Autodesk Fusion 360 part; units mm, degrees
(part 9 of 20)
  spline S703 degree 3 poles (18.7258, -338.1357) (18.7536, -338.279) (18.8048, -338.5439) (18.9786, -338.7491) (19.0584, -338.8434) knots 0 0 0 0 0.042908 0.079365 0.079365 0.079365 0.079365
  spline S704 degree 3 poles (19.0584, -338.8434) (19.1506, -338.9125) (19.3372, -339.0525) (19.5699, -339.0711) (19.6877, -339.0804) knots 0 0 0 0 0.033826 0.068485 0.068485 0.068485 0.068485
  spline S705 degree 3 poles (19.6877, -339.0804) (19.8301, -339.0661) (20.1169, -339.0374) (20.3305, -338.8437) (20.438, -338.7462) knots 0 0 0 0 0.041772 0.0841 0.0841 0.0841 0.0841
  spline S706 degree 3 poles (20.438, -338.7462) (20.5275, -338.6211) (20.7167, -338.3566) (20.7352, -338.031) (20.7449, -337.8594) knots 0 0 0 0 0.045186 0.095569 0.095569 0.095569 0.095569
  spline S707 degree 3 poles (20.7449, -337.8594) (20.7359, -337.6971) (20.7188, -337.3908) (20.5359, -337.1458) (20.4499, -337.0306) knots 0 0 0 0 0.047557 0.089725 0.089725 0.089725 0.089725
  spline S708 degree 3 poles (20.4499, -337.0306) (20.3414, -336.9421) (20.1168, -336.7589) (19.8271, -336.7379) (19.6774, -336.7271) knots 0 0 0 0 0.040971 0.08482 0.08482 0.08482 0.08482
  spline S709 degree 3 poles (19.6774, -336.7271) (19.5817, -336.7322) (19.3944, -336.7423) (19.2249, -336.8225) (19.1419, -336.8618) knots 0 0 0 0 0.028423 0.055689 0.055689 0.055689 0.055689
  spline S710 degree 3 poles (19.1419, -336.8618) (19.0671, -336.9094) (18.9202, -337.0026) (18.8172, -337.1427) (18.7667, -337.2114) knots 0 0 0 0 0.026342 0.051681 0.051681 0.051681 0.051681
  line L196 (18.7667, -337.2114) -> (18.1903, -337.1364)
  line L197 (18.1903, -337.1364) -> (18.6746, -334.5682)
  line L198 (18.6746, -334.5682) -> (21.161, -334.5681)
  line L199 (21.161, -334.5681) -> (21.161, -335.1548)
  line L200 (21.161, -335.1548) -> (19.1657, -335.1548)
  line L201 (19.1657, -335.1548) -> (18.8963, -336.4986)
  spline S711 degree 3 poles (18.8963, -336.4986) (19.0458, -336.4071) (19.3367, -336.2291) (19.6761, -336.1993) (19.8411, -336.1848) knots 0 0 0 0 0.051785 0.100763 0.100763 0.100763 0.100763
  spline S712 degree 3 poles (19.8411, -336.1848) (20.0503, -336.2032) (20.4659, -336.2397) (20.7868, -336.5061) (20.9461, -336.6384) knots 0 0 0 0 0.061424 0.122014 0.122014 0.122014 0.122014
  spline S713 degree 3 poles (20.9461, -336.6384) (21.0774, -336.8038) (21.3483, -337.1451) (21.38, -337.5805) (21.3964, -337.8048) knots 0 0 0 0 0.061868 0.12764 0.12764 0.12764 0.12764
  spline S714 degree 3 poles (21.3964, -337.8048) (21.3812, -338.0218) (21.3513, -338.4476) (21.1161, -338.8035) (21.0008, -338.9781) knots 0 0 0 0 0.064036 0.125703 0.125703 0.125703 0.125703
  spline S715 degree 3 poles (21.0008, -338.9781) (20.823, -339.1551) (20.46, -339.5168) (19.9487, -339.5621) (19.6877, -339.5852) knots 0 0 0 0 0.072854 0.148822 0.148822 0.148822 0.148822
  spline S716 degree 3 poles (19.6877, -339.5852) (19.4745, -339.5725) (19.0669, -339.5481) (18.7332, -339.3146) (18.5741, -339.2033) knots 0 0 0 0 0.062678 0.119794 0.119794 0.119794 0.119794
  spline S717 degree 3 poles (18.5741, -339.2033) (18.4455, -339.0629) (18.1812, -338.7745) (18.1151, -338.3885) (18.0812, -338.1903) knots 0 0 0 0 0.055877 0.114795 0.114795 0.114795 0.114795
  line L202 (29.6139, -389.4998) -> (29.6138, -385.8777)
  line L203 (29.6138, -385.8777) -> (30.163, -385.8777)
  line L204 (30.163, -385.8777) -> (30.163, -386.3859)
  spline S718 degree 3 poles (30.163, -386.3859) (30.2249, -386.3013) (30.3497, -386.1308) (30.5271, -386.0158) (30.6166, -385.9579) knots 0 0 0 0 0.031158 0.062835 0.062835 0.062835 0.062835
  spline S719 degree 3 poles (30.6166, -385.9579) (30.7157, -385.9106) (30.9196, -385.8135) (31.1453, -385.8018) (31.2612, -385.7958) knots 0 0 0 0 0.032617 0.067048 0.067048 0.067048 0.067048
  spline S720 degree 3 poles (31.2612, -385.7958) (31.3857, -385.8006) (31.6181, -385.8094) (31.825, -385.9143) (31.9211, -385.963) knots 0 0 0 0 0.036859 0.068796 0.068796 0.068796 0.068796
  spline S721 degree 3 poles (31.9211, -385.963) (32.0008, -386.0247) (32.1617, -386.1493) (32.2432, -386.336) (32.2844, -386.4302) knots 0 0 0 0 0.029725 0.060035 0.060035 0.060035 0.060035
  spline S722 degree 3 poles (32.2844, -386.4302) (32.4346, -386.2452) (32.7257, -385.8867) (33.1821, -385.8254) (33.4031, -385.7958) knots 0 0 0 0 0.068625 0.133023 0.133023 0.133023 0.133023
  spline S723 degree 3 poles (33.4031, -385.7958) (33.5681, -385.8042) (33.876, -385.8199) (34.1191, -386.0073) (34.2319, -386.0942) knots 0 0 0 0 0.048244 0.08997 0.08997 0.08997 0.08997
  spline S724 degree 3 poles (34.2319, -386.0942) (34.3161, -386.2166) (34.5056, -386.4915) (34.516, -386.8271) (34.5218, -387.0134) knots 0 0 0 0 0.043695 0.098195 0.098195 0.098195 0.098195
  line L205 (34.5218, -387.0134) -> (34.5218, -389.4997)
  line L206 (34.5218, -389.4997) -> (33.9113, -389.4998)
  line L207 (33.9113, -389.4998) -> (33.9113, -387.218)
  spline S725 degree 3 poles (33.9113, -387.218) (33.9112, -387.1118) (33.9112, -386.9325) (33.8688, -386.7586) (33.8516, -386.6877) knots 0 0 0 0 0.031711 0.053535 0.053535 0.053535 0.053535
  spline S726 degree 3 poles (33.8516, -386.6877) (33.8271, -386.636) (33.7773, -386.5306) (33.683, -386.4618) (33.635, -386.4268) knots 0 0 0 0 0.016863 0.034394 0.034394 0.034394 0.034394
  spline S727 degree 3 poles (33.635, -386.4268) (33.5793, -386.3979) (33.4638, -386.3382) (33.3339, -386.3314) (33.2666, -386.3279) knots 0 0 0 0 0.018597 0.038532 0.038532 0.038532 0.038532
  spline S728 degree 3 poles (33.2666, -386.3279) (33.1455, -386.3377) (32.9075, -386.3569) (32.7229, -386.5079) (32.6323, -386.582) knots 0 0 0 0 0.035532 0.069798 0.069798 0.069798 0.069798
  spline S729 degree 3 poles (32.6323, -386.582) (32.5589, -386.6887) (32.3918, -386.9318) (32.3842, -387.2288) (32.3799, -387.3954) knots 0 0 0 0 0.038079 0.086792 0.086792 0.086792 0.086792
  line L208 (32.3799, -387.3954) -> (32.3799, -389.4998)
  line L209 (32.3799, -389.4998) -> (31.766, -389.4998)
  line L210 (31.766, -389.4998) -> (31.766, -387.1464)
  spline S730 degree 3 poles (31.766, -387.1464) (31.7636, -387.0244) (31.7593, -386.8076) (31.6595, -386.6162) (31.6159, -386.5325) knots 0 0 0 0 0.036008 0.063954 0.063954 0.063954 0.063954
  spline S731 degree 3 poles (31.6159, -386.5325) (31.5537, -386.473) (31.4175, -386.3426) (31.2278, -386.3331) (31.1248, -386.3279) knots 0 0 0 0 0.025037 0.054812 0.054812 0.054812 0.054812
  spline S732 degree 3 poles (31.1248, -386.3279) (31.04, -386.3336) (30.8706, -386.3449) (30.7205, -386.4245) (30.6456, -386.4643) knots 0 0 0 0 0.025172 0.050327 0.050327 0.050327 0.050327
  spline S733 degree 3 poles (30.6456, -386.4643) (30.5769, -386.516) (30.4366, -386.6216) (30.3639, -386.7816) (30.3267, -386.8634) knots 0 0 0 0 0.025339 0.051812 0.051812 0.051812 0.051812
  spline S734 degree 3 poles (30.3267, -386.8634) (30.298, -386.9697) (30.2311, -387.2172) (30.229, -387.474) (30.2278, -387.6205) knots 0 0 0 0 0.032907 0.076633 0.076633 0.076633 0.076633
  line L211 (30.2278, -387.6205) -> (30.2278, -389.4998)
  line L212 (30.2278, -389.4998) -> (29.6139, -389.4998)
  line L213 (20.1494, -389.5) -> (20.1493, -388.3028)
  line L214 (20.1493, -388.3028) -> (17.9802, -388.3029)
  line L215 (17.9802, -388.3029) -> (17.9802, -387.7401)
  line L216 (17.9802, -387.7401) -> (20.2618, -384.5)
  line L217 (20.2618, -384.5) -> (20.7632, -384.5)
  line L218 (20.7632, -384.5) -> (20.7633, -387.7401)
  line L219 (20.7633, -387.7401) -> (21.4386, -387.7401)
  line L220 (21.4386, -387.7401) -> (21.4386, -388.3028)
  line L221 (21.4386, -388.3028) -> (20.7633, -388.3028)
  line L222 (20.7633, -388.3028) -> (20.7633, -389.5)
  line L223 (20.7633, -389.5) -> (20.1494, -389.5)
  line L224 (29.6186, -439.4991) -> (29.6184, -435.877)
  line L225 (29.6184, -435.877) -> (30.1675, -435.8769)
  line L226 (30.1675, -435.8769) -> (30.1675, -436.3851)
  spline S735 degree 3 poles (30.1675, -436.3851) (30.2294, -436.3005) (30.3543, -436.13) (30.5317, -436.015) (30.6211, -435.957) knots 0 0 0 0 0.031158 0.062835 0.062835 0.062835 0.062835
  spline S736 degree 3 poles (30.6211, -435.957) (30.7203, -435.9098) (30.9241, -435.8127) (31.1498, -435.801) (31.2657, -435.795) knots 0 0 0 0 0.032617 0.067048 0.067048 0.067048 0.067048
  spline S737 degree 3 poles (31.2657, -435.795) (31.3902, -435.7997) (31.6226, -435.8085) (31.8296, -435.9134) (31.9257, -435.962) knots 0 0 0 0 0.036859 0.068796 0.068796 0.068796 0.068796
  spline S738 degree 3 poles (31.9257, -435.962) (32.0053, -436.0238) (32.1663, -436.1484) (32.2478, -436.3351) (32.2889, -436.4293) knots 0 0 0 0 0.029725 0.060035 0.060035 0.060035 0.060035
  spline S739 degree 3 poles (32.2889, -436.4293) (32.4391, -436.2443) (32.7302, -435.8857) (33.1866, -435.8245) (33.4076, -435.7948) knots 0 0 0 0 0.068625 0.133023 0.133023 0.133023 0.133023
  spline S740 degree 3 poles (33.4076, -435.7948) (33.5727, -435.8032) (33.8805, -435.8189) (34.1236, -436.0063) (34.2364, -436.0932) knots 0 0 0 0 0.048244 0.08997 0.08997 0.08997 0.08997
  spline S741 degree 3 poles (34.2364, -436.0932) (34.3207, -436.2155) (34.5101, -436.4904) (34.5206, -436.826) (34.5264, -437.0123) knots 0 0 0 0 0.043695 0.098195 0.098195 0.098195 0.098195
  line L227 (34.5264, -437.0123) -> (34.5265, -439.4987)
  line L228 (34.5265, -439.4987) -> (33.916, -439.4987)
  line L229 (33.916, -439.4987) -> (33.9159, -437.217)
  spline S742 degree 3 poles (33.9159, -437.217) (33.9158, -437.1108) (33.9158, -436.9315) (33.8734, -436.7576) (33.8561, -436.6867) knots 0 0 0 0 0.031711 0.053535 0.053535 0.053535 0.053535
  spline S743 degree 3 poles (33.8561, -436.6867) (33.8317, -436.635) (33.7819, -436.5296) (33.6876, -436.4608) (33.6395, -436.4258) knots 0 0 0 0 0.016863 0.034394 0.034394 0.034394 0.034394
  spline S744 degree 3 poles (33.6395, -436.4258) (33.5838, -436.3969) (33.4684, -436.3372) (33.3384, -436.3304) (33.2712, -436.3269) knots 0 0 0 0 0.018597 0.038532 0.038532 0.038532 0.038532
  spline S745 degree 3 poles (33.2712, -436.3269) (33.15, -436.3367) (32.9121, -436.356) (32.7275, -436.5069) (32.6368, -436.581) knots 0 0 0 0 0.035532 0.069798 0.069798 0.069798 0.069798
  spline S746 degree 3 poles (32.6368, -436.581) (32.5635, -436.6877) (32.3964, -436.9309) (32.3888, -437.2278) (32.3845, -437.3945) knots 0 0 0 0 0.038079 0.086792 0.086792 0.086792 0.086792
  line L230 (32.3845, -437.3945) -> (32.3847, -439.4988)
  line L231 (32.3847, -439.4988) -> (31.7707, -439.4989)
  line L232 (31.7707, -439.4989) -> (31.7706, -437.1455)
  spline S747 degree 3 poles (31.7706, -437.1455) (31.7681, -437.0235) (31.7638, -436.8067) (31.6641, -436.6153) (31.6205, -436.5316) knots 0 0 0 0 0.036008 0.063954 0.063954 0.063954 0.063954
  spline S748 degree 3 poles (31.6205, -436.5316) (31.5582, -436.4721) (31.422, -436.3417) (31.2323, -436.3322) (31.1293, -436.327) knots 0 0 0 0 0.025037 0.054812 0.054812 0.054812 0.054812
  spline S749 degree 3 poles (31.1293, -436.327) (31.0445, -436.3327) (30.8751, -436.3441) (30.7251, -436.4237) (30.6501, -436.4635) knots 0 0 0 0 0.025172 0.050327 0.050327 0.050327 0.050327
  spline S750 degree 3 poles (30.6501, -436.4635) (30.5815, -436.5152) (30.4412, -436.6208) (30.3684, -436.7808) (30.3313, -436.8626) knots 0 0 0 0 0.025339 0.051812 0.051812 0.051812 0.051812
  spline S751 degree 3 poles (30.3313, -436.8626) (30.3026, -436.9689) (30.2357, -437.2164) (30.2336, -437.4732) (30.2324, -437.6197) knots 0 0 0 0 0.032907 0.076633 0.076633 0.076633 0.076633
  line L233 (30.2324, -437.6197) -> (30.2325, -439.499)
  line L234 (30.2325, -439.499) -> (29.6186, -439.4991)
  line L235 (20.1541, -439.4998) -> (20.154, -438.3027)
  line L236 (20.154, -438.3027) -> (17.9848, -438.3028)
  line L237 (17.9848, -438.3028) -> (17.9848, -437.7401)
  line L238 (17.9848, -437.7401) -> (20.2663, -434.4998)
  line L239 (20.2663, -434.4998) -> (20.7676, -434.4997)
  line L240 (20.7676, -434.4997) -> (20.7679, -437.7398)
  line L241 (20.7679, -437.7398) -> (21.4432, -437.7398)
  line L242 (21.4432, -437.7398) -> (21.4432, -438.3026)
  line L243 (21.4432, -438.3026) -> (20.7679, -438.3026)
  line L244 (20.7679, -438.3026) -> (20.768, -439.4997)
  line L245 (20.768, -439.4997) -> (20.1541, -439.4998)
  line L246 (29.5119, -489.4998) -> (29.5118, -485.8777)
  line L247 (29.5118, -485.8777) -> (30.0609, -485.8777)
  line L248 (30.0609, -485.8777) -> (30.0609, -486.3859)
  spline S752 degree 3 poles (30.0609, -486.3859) (30.1228, -486.3013) (30.2477, -486.1308) (30.4251, -486.0158) (30.5145, -485.9579) knots 0 0 0 0 0.031158 0.062835 0.062835 0.062835 0.062835
  spline S753 degree 3 poles (30.5145, -485.9579) (30.6137, -485.9106) (30.8176, -485.8135) (31.0433, -485.8018) (31.1591, -485.7958) knots 0 0 0 0 0.032617 0.067048 0.067048 0.067048 0.067048
  spline S754 degree 3 poles (31.1591, -485.7958) (31.2836, -485.8006) (31.516, -485.8094) (31.723, -485.9143) (31.8191, -485.9629) knots 0 0 0 0 0.036859 0.068796 0.068796 0.068796 0.068796
  spline S755 degree 3 poles (31.8191, -485.9629) (31.8988, -486.0247) (32.0597, -486.1493) (32.1412, -486.336) (32.1824, -486.4302) knots 0 0 0 0 0.029725 0.060035 0.060035 0.060035 0.060035
  spline S756 degree 3 poles (32.1824, -486.4302) (32.3325, -486.2452) (32.6236, -485.8867) (33.0801, -485.8254) (33.301, -485.7958) knots 0 0 0 0 0.068625 0.133023 0.133023 0.133023 0.133023
  spline S757 degree 3 poles (33.301, -485.7958) (33.4661, -485.8042) (33.774, -485.8199) (34.0171, -486.0073) (34.1298, -486.0942) knots 0 0 0 0 0.048244 0.08997 0.08997 0.08997 0.08997
  spline S758 degree 3 poles (34.1298, -486.0942) (34.2141, -486.2165) (34.4035, -486.4914) (34.414, -486.8271) (34.4197, -487.0134) knots 0 0 0 0 0.043695 0.098195 0.098195 0.098195 0.098195
  line L249 (34.4197, -487.0134) -> (34.4198, -489.4997)
  line L250 (34.4198, -489.4997) -> (33.8093, -489.4998)
  line L251 (33.8093, -489.4998) -> (33.8092, -487.218)
  spline S759 degree 3 poles (33.8092, -487.218) (33.8092, -487.1118) (33.8092, -486.9325) (33.7668, -486.7586) (33.7495, -486.6877) knots 0 0 0 0 0.031711 0.053535 0.053535 0.053535 0.053535
  spline S760 degree 3 poles (33.7495, -486.6877) (33.7251, -486.636) (33.6753, -486.5306) (33.581, -486.4618) (33.533, -486.4268) knots 0 0 0 0 0.016863 0.034394 0.034394 0.034394 0.034394
  spline S761 degree 3 poles (33.533, -486.4268) (33.4772, -486.3979) (33.3618, -486.3382) (33.2318, -486.3314) (33.1646, -486.3279) knots 0 0 0 0 0.018597 0.038532 0.038532 0.038532 0.038532
  spline S762 degree 3 poles (33.1646, -486.3279) (33.0435, -486.3377) (32.8055, -486.3569) (32.6209, -486.5079) (32.5302, -486.582) knots 0 0 0 0 0.035532 0.069798 0.069798 0.069798 0.069798
  spline S763 degree 3 poles (32.5302, -486.582) (32.4569, -486.6887) (32.2898, -486.9318) (32.2821, -487.2288) (32.2779, -487.3954) knots 0 0 0 0 0.038079 0.086792 0.086792 0.086792 0.086792
  line L252 (32.2779, -487.3954) -> (32.2779, -489.4998)
  line L253 (32.2779, -489.4998) -> (31.664, -489.4998)
  line L254 (31.664, -489.4998) -> (31.6639, -487.1464)
  spline S764 degree 3 poles (31.6639, -487.1464) (31.6615, -487.0244) (31.6572, -486.8076) (31.5575, -486.6162) (31.5139, -486.5325) knots 0 0 0 0 0.036008 0.063954 0.063954 0.063954 0.063954
  spline S765 degree 3 poles (31.5139, -486.5325) (31.4516, -486.473) (31.3154, -486.3426) (31.1258, -486.3331) (31.0227, -486.3279) knots 0 0 0 0 0.025037 0.054812 0.054812 0.054812 0.054812
  spline S766 degree 3 poles (31.0227, -486.3279) (30.938, -486.3336) (30.7685, -486.3449) (30.6185, -486.4245) (30.5435, -486.4643) knots 0 0 0 0 0.025173 0.050327 0.050327 0.050327 0.050327
  spline S767 degree 3 poles (30.5435, -486.4643) (30.4749, -486.516) (30.3346, -486.6216) (30.2618, -486.7816) (30.2246, -486.8634) knots 0 0 0 0 0.025339 0.051812 0.051812 0.051812 0.051812
  spline S768 degree 3 poles (30.2246, -486.8634) (30.1959, -486.9697) (30.1291, -487.2172) (30.127, -487.474) (30.1258, -487.6205) knots 0 0 0 0 0.032907 0.076633 0.076633 0.076633 0.076633
  line L255 (30.1258, -487.6205) -> (30.1258, -489.4998)
  line L256 (30.1258, -489.4998) -> (29.5119, -489.4998)
  line L257 (18.0828, -488.1801) -> (18.6967, -488.0982)
  spline S769 degree 3 poles (18.6967, -488.0982) (18.7321, -488.254) (18.7955, -488.533) (18.9765, -488.7531) (19.0565, -488.8503) knots 0 0 0 0 0.04711 0.084389 0.084389 0.084389 0.084389
  spline S770 degree 3 poles (19.0565, -488.8503) (19.1469, -488.9174) (19.3307, -489.054) (19.5593, -489.0716) (19.6756, -489.0805) knots 0 0 0 0 0.033049 0.06726 0.06726 0.06726 0.06726
  spline S771 degree 3 poles (19.6756, -489.0805) (19.814, -489.0683) (20.0891, -489.0441) (20.3016, -488.8679) (20.4071, -488.7803) knots 0 0 0 0 0.040646 0.080767 0.080767 0.080767 0.080767
  spline S772 degree 3 poles (20.4071, -488.7803) (20.4942, -488.6734) (20.6706, -488.4566) (20.6938, -488.1779) (20.7056, -488.0368) knots 0 0 0 0 0.040368 0.081802 0.081802 0.081802 0.081802
  spline S773 degree 3 poles (20.7056, -488.0368) (20.6952, -487.9031) (20.6748, -487.6418) (20.5099, -487.4386) (20.4293, -487.3393) knots 0 0 0 0 0.039196 0.07662 0.07662 0.07662 0.07662
  spline S774 degree 3 poles (20.4293, -487.3393) (20.3292, -487.2593) (20.1239, -487.095) (19.8613, -487.075) (19.7267, -487.0648) knots 0 0 0 0 0.037531 0.077014 0.077014 0.077014 0.077014
  spline S775 degree 3 poles (19.7267, -487.0648) (19.6613, -487.0687) (19.5148, -487.0774) (19.3724, -487.1132) (19.2935, -487.133) knots 0 0 0 0 0.0196 0.043933 0.043933 0.043933 0.043933
  line L258 (19.2935, -487.133) -> (19.3618, -486.5941)
  spline S776 degree 3 poles (19.3618, -486.5941) (19.3802, -486.5961) (19.4131, -486.5996) (19.4462, -486.6005) (19.4607, -486.6009) knots 0 0 0 0 0.005566 0.009918 0.009918 0.009918 0.009918
  spline S777 degree 3 poles (19.4607, -486.6009) (19.5875, -486.5928) (19.838, -486.5768) (20.058, -486.456) (20.1667, -486.3963) knots 0 0 0 0 0.037611 0.074313 0.074313 0.074313 0.074313
  spline S778 degree 3 poles (20.1667, -486.3963) (20.2581, -486.3162) (20.4485, -486.1497) (20.4695, -485.8967) (20.4804, -485.7653) knots 0 0 0 0 0.035073 0.072985 0.072985 0.072985 0.072985
  spline S779 degree 3 poles (20.4804, -485.7653) (20.4716, -485.6582) (20.4541, -485.4476) (20.3186, -485.2856) (20.2519, -485.206) knots 0 0 0 0 0.031391 0.061757 0.061757 0.061757 0.061757
  spline S780 degree 3 poles (20.2519, -485.206) (20.1682, -485.1413) (19.9946, -485.0073) (19.7754, -484.9921) (19.6619, -484.9843) knots 0 0 0 0 0.031011 0.064303 0.064303 0.064303 0.064303
  spline S781 degree 3 poles (19.6619, -484.9843) (19.5485, -484.9927) (19.3271, -485.0092) (19.1509, -485.1438) (19.065, -485.2094) knots 0 0 0 0 0.033306 0.06503 0.06503 0.06503 0.06503
  spline S782 degree 3 poles (19.065, -485.2094) (18.9918, -485.2995) (18.8312, -485.4971) (18.7838, -485.7481) (18.7581, -485.8847) knots 0 0 0 0 0.034298 0.07522 0.07522 0.07522 0.07522
  line L259 (18.7581, -485.8847) -> (18.1441, -485.7756)
  spline S783 degree 3 poles (18.1441, -485.7756) (18.19, -485.5845) (18.2776, -485.2203) (18.5339, -484.9482) (18.6557, -484.8189) knots 0 0 0 0 0.057796 0.110176 0.110176 0.110176 0.110176
  spline S784 degree 3 poles (18.6557, -484.8189) (18.8, -484.7199) (19.0988, -484.515) (19.461, -484.4916) (19.6482, -484.4795) knots 0 0 0 0 0.051494 0.106636 0.106636 0.106636 0.106636
  spline S785 degree 3 poles (19.6482, -484.4795) (19.7811, -484.4864) (20.0429, -484.4999) (20.2835, -484.6039) (20.402, -484.6551) knots 0 0 0 0 0.039552 0.07795 0.07795 0.07795 0.07795
  spline S786 degree 3 poles (20.402, -484.6551) (20.5093, -484.7178) (20.7191, -484.8402) (20.8601, -485.0378) (20.9289, -485.1343) knots 0 0 0 0 0.036811 0.071949 0.071949 0.071949 0.071949
  spline S787 degree 3 poles (20.9289, -485.1343) (20.9821, -485.2365) (21.0875, -485.4388) (21.1035, -485.6663) (21.1114, -485.7789) knots 0 0 0 0 0.034154 0.067635 0.067635 0.067635 0.067635
  spline S788 degree 3 poles (21.1114, -485.7789) (21.1043, -485.8843) (21.0902, -486.0939) (20.9882, -486.2776) (20.9375, -486.369) knots 0 0 0 0 0.031256 0.062193 0.062193 0.062193 0.062193
  spline S789 degree 3 poles (20.9375, -486.369) (20.8702, -486.4542) (20.7295, -486.6323) (20.5278, -486.7372) (20.4225, -486.7919) knots 0 0 0 0 0.032177 0.067318 0.067318 0.067318 0.067318
  spline S790 degree 3 poles (20.4225, -486.7919) (20.5606, -486.8334) (20.8284, -486.9138) (21.0191, -487.1178) (21.1114, -487.2165) knots 0 0 0 0 0.042418 0.082229 0.082229 0.082229 0.082229
  spline S791 degree 3 poles (21.1114, -487.2165) (21.183, -487.3343) (21.3334, -487.5817) (21.3489, -487.8713) (21.357, -488.0231) knots 0 0 0 0 0.040688 0.085491 0.085491 0.085491 0.085491
  spline S792 degree 3 poles (21.357, -488.0231) (21.3369, -488.2333) (21.2967, -488.6544) (21.0188, -488.9735) (20.8795, -489.1333) knots 0 0 0 0 0.061663 0.123588 0.123588 0.123588 0.123588
  spline S793 degree 3 poles (20.8795, -489.1333) (20.7066, -489.2661) (20.3507, -489.5393) (19.9026, -489.5719) (19.6722, -489.5886) knots 0 0 0 0 0.063941 0.131584 0.131584 0.131584 0.131584
  spline S794 degree 3 poles (19.6722, -489.5886) (19.4646, -489.5745) (19.0624, -489.5472) (18.7367, -489.3108) (18.5791, -489.1964) knots 0 0 0 0 0.061033 0.118246 0.118246 0.118246 0.118246
  spline S795 degree 3 poles (18.5791, -489.1964) (18.4495, -489.0541) (18.1853, -488.764) (18.1174, -488.3772) (18.0828, -488.1801) knots 0 0 0 0 0.056507 0.1152 0.1152 0.1152 0.1152
  line L260 (29.5184, -539.499) -> (29.5181, -535.8769)
  line L261 (29.5181, -535.8769) -> (30.0672, -535.8768)
  line L262 (30.0672, -535.8768) -> (30.0672, -536.385)
  spline S796 degree 3 poles (30.0672, -536.385) (30.1291, -536.3004) (30.254, -536.1299) (30.4314, -536.0149) (30.5208, -535.9569) knots 0 0 0 0 0.031158 0.062835 0.062835 0.062835 0.062835
  spline S797 degree 3 poles (30.5208, -535.9569) (30.62, -535.9097) (30.8239, -535.8125) (31.0495, -535.8009) (31.1654, -535.7949) knots 0 0 0 0 0.032617 0.067048 0.067048 0.067048 0.067048
  spline S798 degree 3 poles (31.1654, -535.7949) (31.2899, -535.7996) (31.5223, -535.8084) (31.7293, -535.9133) (31.8254, -535.9619) knots 0 0 0 0 0.036859 0.068796 0.068796 0.068796 0.068796
  spline S799 degree 3 poles (31.8254, -535.9619) (31.9051, -536.0236) (32.066, -536.1483) (32.1475, -536.3349) (32.1887, -536.4291) knots 0 0 0 0 0.029725 0.060035 0.060035 0.060035 0.060035
  spline S800 degree 3 poles (32.1887, -536.4291) (32.3388, -536.2442) (32.6299, -535.8856) (33.0863, -535.8243) (33.3073, -535.7947) knots 0 0 0 0 0.068625 0.133023 0.133023 0.133023 0.133023
  spline S801 degree 3 poles (33.3073, -535.7947) (33.4724, -535.8031) (33.7803, -535.8187) (34.0234, -536.0061) (34.1361, -536.093) knots 0 0 0 0 0.048244 0.08997 0.08997 0.08997 0.08997
  spline S802 degree 3 poles (34.1361, -536.093) (34.2204, -536.2154) (34.4099, -536.4902) (34.4203, -536.8259) (34.4261, -537.0122) knots 0 0 0 0 0.043695 0.098195 0.098195 0.098195 0.098195
  line L263 (34.4261, -537.0122) -> (34.4263, -539.4985)
  line L264 (34.4263, -539.4985) -> (33.8158, -539.4986)
  line L265 (33.8158, -539.4986) -> (33.8156, -537.2169)
  spline S803 degree 3 poles (33.8156, -537.2169) (33.8156, -537.1106) (33.8155, -536.9313) (33.7731, -536.7574) (33.7559, -536.6865) knots 0 0 0 0 0.031711 0.053535 0.053535 0.053535 0.053535
  spline S804 degree 3 poles (33.7559, -536.6865) (33.7314, -536.6348) (33.6816, -536.5294) (33.5873, -536.4607) (33.5393, -536.4256) knots 0 0 0 0 0.016863 0.034394 0.034394 0.034394 0.034394
  spline S805 degree 3 poles (33.5393, -536.4256) (33.4836, -536.3968) (33.3681, -536.337) (33.2381, -536.3303) (33.1709, -536.3267) knots 0 0 0 0 0.018597 0.038532 0.038532 0.038532 0.038532
  spline S806 degree 3 poles (33.1709, -536.3267) (33.0498, -536.3366) (32.8118, -536.3558) (32.6272, -536.5068) (32.5366, -536.5809) knots 0 0 0 0 0.035532 0.069798 0.069798 0.069798 0.069798
  spline S807 degree 3 poles (32.5366, -536.5809) (32.4632, -536.6876) (32.2961, -536.9308) (32.2885, -537.2277) (32.2842, -537.3944) knots 0 0 0 0 0.038079 0.086792 0.086792 0.086792 0.086792
  line L266 (32.2842, -537.3944) -> (32.2844, -539.4987)
  line L267 (32.2844, -539.4987) -> (31.6705, -539.4988)
  line L268 (31.6705, -539.4988) -> (31.6703, -537.1454)
  spline S808 degree 3 poles (31.6703, -537.1454) (31.6679, -537.0234) (31.6636, -536.8066) (31.5638, -536.6152) (31.5202, -536.5315) knots 0 0 0 0 0.036008 0.063954 0.063954 0.063954 0.063954
  spline S809 degree 3 poles (31.5202, -536.5315) (31.458, -536.472) (31.3217, -536.3416) (31.1321, -536.3321) (31.029, -536.3269) knots 0 0 0 0 0.025037 0.054812 0.054812 0.054812 0.054812
  spline S810 degree 3 poles (31.029, -536.3269) (30.9443, -536.3326) (30.7748, -536.344) (30.6248, -536.4236) (30.5499, -536.4634) knots 0 0 0 0 0.025173 0.050327 0.050327 0.050327 0.050327
  spline S811 degree 3 poles (30.5499, -536.4634) (30.4812, -536.5151) (30.3409, -536.6207) (30.2682, -536.7807) (30.231, -536.8625) knots 0 0 0 0 0.025339 0.051812 0.051812 0.051812 0.051812
  spline S812 degree 3 poles (30.231, -536.8625) (30.2023, -536.9688) (30.1355, -537.2163) (30.1334, -537.4731) (30.1321, -537.6196) knots 0 0 0 0 0.032907 0.076633 0.076633 0.076633 0.076633
  line L269 (30.1321, -537.6196) -> (30.1323, -539.4989)
  line L270 (30.1323, -539.4989) -> (29.5184, -539.499)
  line L271 (18.0892, -538.18) -> (18.7031, -538.0981)
  spline S813 degree 3 poles (18.7031, -538.0981) (18.7385, -538.2539) (18.8019, -538.5329) (18.983, -538.7529) (19.063, -538.8501) knots 0 0 0 0 0.04711 0.084389 0.084389 0.084389 0.084389
  spline S814 degree 3 poles (19.063, -538.8501) (19.1534, -538.9173) (19.3372, -539.0539) (19.5658, -539.0714) (19.6821, -539.0803) knots 0 0 0 0 0.033049 0.06726 0.06726 0.06726 0.06726
  spline S815 degree 3 poles (19.6821, -539.0803) (19.8205, -539.0681) (20.0956, -539.0439) (20.3081, -538.8676) (20.4136, -538.7801) knots 0 0 0 0 0.040646 0.080767 0.080767 0.080767 0.080767
  spline S816 degree 3 poles (20.4136, -538.7801) (20.5007, -538.6731) (20.677, -538.4564) (20.7002, -538.1777) (20.712, -538.0365) knots 0 0 0 0 0.040368 0.081802 0.081802 0.081802 0.081802
  spline S817 degree 3 poles (20.712, -538.0365) (20.7016, -537.9029) (20.6812, -537.6416) (20.5162, -537.4384) (20.4357, -537.3391) knots 0 0 0 0 0.039196 0.07662 0.07662 0.07662 0.07662
  spline S818 degree 3 poles (20.4357, -537.3391) (20.3356, -537.259) (20.1303, -537.0948) (19.8677, -537.0748) (19.7331, -537.0646) knots 0 0 0 0 0.037531 0.077014 0.077014 0.077014 0.077014
  spline S819 degree 3 poles (19.7331, -537.0646) (19.6677, -537.0685) (19.5212, -537.0772) (19.3788, -537.113) (19.2999, -537.1328) knots 0 0 0 0 0.0196 0.043933 0.043933 0.043933 0.043933
  line L272 (19.2999, -537.1328) -> (19.3681, -536.594)
  spline S820 degree 3 poles (19.3681, -536.594) (19.3865, -536.5959) (19.4194, -536.5995) (19.4525, -536.6004) (19.467, -536.6008) knots 0 0 0 0 0.005566 0.009918 0.009918 0.009918 0.009918
  spline S821 degree 3 poles (19.467, -536.6008) (19.5938, -536.5927) (19.8444, -536.5766) (20.0643, -536.4558) (20.173, -536.3961) knots 0 0 0 0 0.037611 0.074313 0.074313 0.074313 0.074313
  spline S822 degree 3 poles (20.173, -536.3961) (20.2644, -536.316) (20.4548, -536.1495) (20.4758, -535.8965) (20.4867, -535.7651) knots 0 0 0 0 0.035073 0.072985 0.072985 0.072985 0.072985
  spline S823 degree 3 poles (20.4867, -535.7651) (20.4778, -535.658) (20.4603, -535.4473) (20.3248, -535.2854) (20.2581, -535.2058) knots 0 0 0 0 0.031391 0.061757 0.061757 0.061757 0.061757
  spline S824 degree 3 poles (20.2581, -535.2058) (20.1744, -535.1411) (20.0008, -535.0071) (19.7816, -534.992) (19.6681, -534.9841) knots 0 0 0 0 0.031011 0.064303 0.064303 0.064303 0.064303
  spline S825 degree 3 poles (19.6681, -534.9841) (19.5547, -534.9926) (19.3333, -535.009) (19.1572, -535.1436) (19.0712, -535.2093) knots 0 0 0 0 0.033306 0.06503 0.06503 0.06503 0.06503
  spline S826 degree 3 poles (19.0712, -535.2093) (18.998, -535.2994) (18.8375, -535.4969) (18.7901, -535.748) (18.7643, -535.8846) knots 0 0 0 0 0.034298 0.07522 0.07522 0.07522 0.07522
  line L273 (18.7643, -535.8846) -> (18.1504, -535.7755)
  spline S827 degree 3 poles (18.1504, -535.7755) (18.1963, -535.5844) (18.2838, -535.2202) (18.5401, -534.9481) (18.6619, -534.8188) knots 0 0 0 0 0.057796 0.110176 0.110176 0.110176 0.110176
  spline S828 degree 3 poles (18.6619, -534.8188) (18.8062, -534.7198) (19.105, -534.5149) (19.4671, -534.4915) (19.6544, -534.4793) knots 0 0 0 0 0.051494 0.106636 0.106636 0.106636 0.106636
  spline S829 degree 3 poles (19.6544, -534.4793) (19.7872, -534.4862) (20.0491, -534.4997) (20.2896, -534.6037) (20.4082, -534.6549) knots 0 0 0 0 0.039552 0.07795 0.07795 0.07795 0.07795
  spline S830 degree 3 poles (20.4082, -534.6549) (20.5155, -534.7176) (20.7253, -534.84) (20.8663, -535.0376) (20.9351, -535.1341) knots 0 0 0 0 0.036811 0.071949 0.071949 0.071949 0.071949
  spline S831 degree 3 poles (20.9351, -535.1341) (20.9884, -535.2362) (21.0938, -535.4385) (21.1098, -535.6661) (21.1177, -535.7787) knots 0 0 0 0 0.034154 0.067635 0.067635 0.067635 0.067635
  spline S832 degree 3 poles (21.1177, -535.7787) (21.1106, -535.884) (21.0965, -536.0937) (20.9945, -536.2774) (20.9438, -536.3687) knots 0 0 0 0 0.031256 0.062193 0.062193 0.062193 0.062193
  spline S833 degree 3 poles (20.9438, -536.3687) (20.8765, -536.4539) (20.7358, -536.6321) (20.5341, -536.7369) (20.4288, -536.7917) knots 0 0 0 0 0.032177 0.067318 0.067318 0.067318 0.067318
  spline S834 degree 3 poles (20.4288, -536.7917) (20.567, -536.8332) (20.8348, -536.9135) (21.0255, -537.1175) (21.1178, -537.2163) knots 0 0 0 0 0.042418 0.082229 0.082229 0.082229 0.082229
  spline S835 degree 3 poles (21.1178, -537.2163) (21.1894, -537.334) (21.3398, -537.5814) (21.3553, -537.871) (21.3634, -538.0228) knots 0 0 0 0 0.040688 0.085491 0.085491 0.085491 0.085491
  spline S836 degree 3 poles (21.3634, -538.0228) (21.3434, -538.233) (21.3032, -538.6541) (21.0253, -538.9732) (20.886, -539.1331) knots 0 0 0 0 0.061663 0.123588 0.123588 0.123588 0.123588
  spline S837 degree 3 poles (20.886, -539.1331) (20.7131, -539.2658) (20.3573, -539.5391) (19.9091, -539.5717) (19.6787, -539.5885) knots 0 0 0 0 0.063941 0.131584 0.131584 0.131584 0.131584
  spline S838 degree 3 poles (19.6787, -539.5885) (19.4711, -539.5744) (19.0689, -539.547) (18.7432, -539.3107) (18.5856, -539.1963) knots 0 0 0 0 0.061033 0.118246 0.118246 0.118246 0.118246
  spline S839 degree 3 poles (18.5856, -539.1963) (18.456, -539.054) (18.1918, -538.7639) (18.1238, -538.3771) (18.0892, -538.18) knots 0 0 0 0 0.056507 0.1152 0.1152 0.1152 0.1152
  line L274 (29.5554, -589.4999) -> (29.5554, -585.8778)
  line L275 (29.5554, -585.8778) -> (30.1045, -585.8778)
  line L276 (30.1045, -585.8778) -> (30.1045, -586.386)
  spline S840 degree 3 poles (30.1045, -586.386) (30.1664, -586.3014) (30.2913, -586.1309) (30.4687, -586.0159) (30.5581, -585.958) knots 0 0 0 0 0.031158 0.062835 0.062835 0.062835 0.062835
  spline S841 degree 3 poles (30.5581, -585.958) (30.6573, -585.9107) (30.8612, -585.8136) (31.0868, -585.802) (31.2027, -585.796) knots 0 0 0 0 0.032617 0.067048 0.067048 0.067048 0.067048
  spline S842 degree 3 poles (31.2027, -585.796) (31.3272, -585.8007) (31.5596, -585.8095) (31.7666, -585.9144) (31.8627, -585.9631) knots 0 0 0 0 0.036859 0.068796 0.068796 0.068796 0.068796
  spline S843 degree 3 poles (31.8627, -585.9631) (31.9424, -586.0248) (32.1033, -586.1495) (32.1848, -586.3361) (32.2259, -586.4303) knots 0 0 0 0 0.029725 0.060035 0.060035 0.060035 0.060035
  spline S844 degree 3 poles (32.2259, -586.4303) (32.3761, -586.2454) (32.6672, -585.8868) (33.1236, -585.8256) (33.3446, -585.796) knots 0 0 0 0 0.068625 0.133023 0.133023 0.133023 0.133023
  spline S845 degree 3 poles (33.3446, -585.796) (33.5097, -585.8044) (33.8176, -585.82) (34.0607, -586.0075) (34.1734, -586.0944) knots 0 0 0 0 0.048244 0.08997 0.08997 0.08997 0.08997
  spline S846 degree 3 poles (34.1734, -586.0944) (34.2577, -586.2167) (34.4471, -586.4916) (34.4575, -586.8273) (34.4633, -587.0135) knots 0 0 0 0 0.043695 0.098195 0.098195 0.098195 0.098195
  line L277 (34.4633, -587.0135) -> (34.4633, -589.4999)
  line L278 (34.4633, -589.4999) -> (33.8528, -589.4999)
  line L279 (33.8528, -589.4999) -> (33.8528, -587.2182)
  spline S847 degree 3 poles (33.8528, -587.2182) (33.8528, -587.112) (33.8527, -586.9327) (33.8104, -586.7587) (33.7931, -586.6878) knots 0 0 0 0 0.031711 0.053535 0.053535 0.053535 0.053535
  spline S848 degree 3 poles (33.7931, -586.6878) (33.7687, -586.6362) (33.7188, -586.5308) (33.6246, -586.462) (33.5765, -586.4269) knots 0 0 0 0 0.016863 0.034394 0.034394 0.034394 0.034394
  spline S849 degree 3 poles (33.5765, -586.4269) (33.5208, -586.3981) (33.4054, -586.3383) (33.2754, -586.3315) (33.2082, -586.328) knots 0 0 0 0 0.018597 0.038532 0.038532 0.038532 0.038532
  spline S850 degree 3 poles (33.2082, -586.328) (33.087, -586.3378) (32.8491, -586.3571) (32.6644, -586.508) (32.5738, -586.5821) knots 0 0 0 0 0.035532 0.069798 0.069798 0.069798 0.069798
  spline S851 degree 3 poles (32.5738, -586.5821) (32.5005, -586.6888) (32.3333, -586.932) (32.3257, -587.2289) (32.3214, -587.3955) knots 0 0 0 0 0.038079 0.086792 0.086792 0.086792 0.086792
  line L280 (32.3214, -587.3955) -> (32.3214, -589.4999)
  line L281 (32.3214, -589.4999) -> (31.7075, -589.4999)
  line L282 (31.7075, -589.4999) -> (31.7075, -587.1466)
  spline S852 degree 3 poles (31.7075, -587.1466) (31.7051, -587.0245) (31.7008, -586.8077) (31.601, -586.6163) (31.5574, -586.5327) knots 0 0 0 0 0.036008 0.063954 0.063954 0.063954 0.063954
  spline S853 degree 3 poles (31.5574, -586.5327) (31.4952, -586.4731) (31.359, -586.3427) (31.1693, -586.3332) (31.0663, -586.328) knots 0 0 0 0 0.025037 0.054812 0.054812 0.054812 0.054812
  spline S854 degree 3 poles (31.0663, -586.328) (30.9815, -586.3337) (30.8121, -586.345) (30.6621, -586.4247) (30.5871, -586.4645) knots 0 0 0 0 0.025172 0.050327 0.050327 0.050327 0.050327
  spline S855 degree 3 poles (30.5871, -586.4645) (30.5185, -586.5161) (30.3782, -586.6217) (30.3054, -586.7817) (30.2682, -586.8635) knots 0 0 0 0 0.025339 0.051812 0.051812 0.051812 0.051812
  spline S856 degree 3 poles (30.2682, -586.8635) (30.2395, -586.9698) (30.1727, -587.2173) (30.1705, -587.4741) (30.1693, -587.6207) knots 0 0 0 0 0.032907 0.076633 0.076633 0.076633 0.076633
  line L283 (30.1693, -587.6207) -> (30.1693, -589.4999)
  line L284 (30.1693, -589.4999) -> (29.5554, -589.4999)
  line L285 (21.3494, -588.9099) -> (21.3494, -589.5)
  line L286 (21.3494, -589.5) -> (18.0445, -589.5)
  spline S857 degree 3 poles (18.0445, -589.5) (18.0457, -589.4269) (18.0482, -589.2812) (18.0935, -589.1427) (18.1161, -589.0737) knots 0 0 0 0 0.021791 0.043448 0.043448 0.043448 0.043448
  spline S858 degree 3 poles (18.1161, -589.0737) (18.1664, -588.9593) (18.2717, -588.7199) (18.435, -588.5154) (18.5203, -588.4086) knots 0 0 0 0 0.037314 0.078118 0.078118 0.078118 0.078118
  spline S859 degree 3 poles (18.5203, -588.4086) (18.6313, -588.2886) (18.8818, -588.0181) (19.1656, -587.7825) (19.3235, -587.6514) knots 0 0 0 0 0.048996 0.110487 0.110487 0.110487 0.110487
  spline S860 degree 3 poles (19.3235, -587.6514) (19.5582, -587.459) (19.9537, -587.1347) (20.2889, -586.7491) (20.4251, -586.5924) knots 0 0 0 0 0.090844 0.153043 0.153043 0.153043 0.153043
  spline S861 degree 3 poles (20.4251, -586.5924) (20.5085, -586.4701) (20.6616, -586.2455) (20.696, -585.9766) (20.7116, -585.854) knots 0 0 0 0 0.043642 0.080205 0.080205 0.080205 0.080205
  spline S862 degree 3 poles (20.7116, -585.854) (20.7008, -585.7372) (20.6793, -585.5042) (20.5268, -585.3268) (20.4507, -585.2384) knots 0 0 0 0 0.034264 0.068363 0.068363 0.068363 0.068363
  spline S863 degree 3 poles (20.4507, -585.2384) (20.3544, -585.1653) (20.1536, -585.0129) (19.9015, -584.9963) (19.7702, -584.9877) knots 0 0 0 0 0.035452 0.073952 0.073952 0.073952 0.073952
  spline S864 degree 3 poles (19.7702, -584.9877) (19.6321, -584.9966) (19.368, -585.0136) (19.16, -585.1762) (19.0608, -585.2537) knots 0 0 0 0 0.040455 0.077352 0.077352 0.077352 0.077352
  spline S865 degree 3 poles (19.0608, -585.2537) (18.9832, -585.3553) (18.8174, -585.572) (18.8004, -585.8453) (18.7914, -585.9904) knots 0 0 0 0 0.037518 0.080034 0.080034 0.080034 0.080034
  line L287 (18.7914, -585.9904) -> (18.1604, -585.9256)
  spline S866 degree 3 poles (18.1604, -585.9256) (18.1919, -585.7089) (18.2511, -585.3018) (18.5216, -584.9937) (18.6481, -584.8496) knots 0 0 0 0 0.064088 0.120417 0.120417 0.120417 0.120417
  spline S867 degree 3 poles (18.6481, -584.8496) (18.8081, -584.7418) (19.1503, -584.5111) (19.5637, -584.4905) (19.7839, -584.4795) knots 0 0 0 0 0.056784 0.121484 0.121484 0.121484 0.121484
  spline S868 degree 3 poles (19.7839, -584.4795) (20.0064, -584.4917) (20.4261, -584.5148) (20.7642, -584.7623) (20.923, -584.8786) knots 0 0 0 0 0.065229 0.123034 0.123034 0.123034 0.123034
  spline S869 degree 3 poles (20.923, -584.8786) (21.0454, -585.02) (21.2914, -585.3046) (21.3255, -585.6793) (21.3426, -585.8676) knots 0 0 0 0 0.054646 0.10988 0.10988 0.10988 0.10988
  spline S870 degree 3 poles (21.3426, -585.8676) (21.3372, -585.9678) (21.3263, -586.1707) (21.2556, -586.3612) (21.2198, -586.4577) knots 0 0 0 0 0.029916 0.060578 0.060578 0.060578 0.060578
  spline S871 degree 3 poles (21.2198, -586.4577) (21.1689, -586.5592) (21.0584, -586.7794) (20.8984, -586.967) (20.8122, -587.0682) knots 0 0 0 0 0.033943 0.073642 0.073642 0.073642 0.073642
  spline S872 degree 3 poles (20.8122, -587.0682) (20.6875, -587.1967) (20.3873, -587.5062) (20.0582, -587.7851) (19.8658, -587.9481) knots 0 0 0 0 0.05369 0.129298 0.129298 0.129298 0.129298
  spline S873 degree 3 poles (19.8658, -587.9481) (19.7127, -588.0758) (19.4698, -588.2784) (19.241, -588.4967) (19.1563, -588.5774) knots 0 0 0 0 0.059772 0.09485 0.09485 0.09485 0.09485
  spline S874 degree 3 poles (19.1563, -588.5774) (19.107, -588.6315) (19.012, -588.7356) (18.9345, -588.8533) (18.8971, -588.9099) knots 0 0 0 0 0.021914 0.042221 0.042221 0.042221 0.042221
  line L288 (18.8971, -588.9099) -> (21.3494, -588.9099)
  line L289 (29.5579, -639.4997) -> (29.5578, -635.8776)
  line L290 (29.5578, -635.8776) -> (30.1069, -635.8775)
  line L291 (30.1069, -635.8775) -> (30.1069, -636.3857)
  spline S875 degree 3 poles (30.1069, -636.3857) (30.1688, -636.3012) (30.2937, -636.1306) (30.4711, -636.0156) (30.5605, -635.9577) knots 0 0 0 0 0.031158 0.062835 0.062835 0.062835 0.062835
  spline S876 degree 3 poles (30.5605, -635.9577) (30.6597, -635.9104) (30.8636, -635.8133) (31.0892, -635.8016) (31.2051, -635.7956) knots 0 0 0 0 0.032617 0.067048 0.067048 0.067048 0.067048
  spline S877 degree 3 poles (31.2051, -635.7956) (31.3296, -635.8004) (31.562, -635.8092) (31.769, -635.9141) (31.8651, -635.9628) knots 0 0 0 0 0.036859 0.068796 0.068796 0.068796 0.068796
  spline S878 degree 3 poles (31.8651, -635.9628) (31.9448, -636.0245) (32.1057, -636.1491) (32.1872, -636.3358) (32.2283, -636.43) knots 0 0 0 0 0.029725 0.060035 0.060035 0.060035 0.060035
  spline S879 degree 3 poles (32.2283, -636.43) (32.3785, -636.245) (32.6696, -635.8865) (33.126, -635.8252) (33.347, -635.7956) knots 0 0 0 0 0.068625 0.133023 0.133023 0.133023 0.133023
  spline S880 degree 3 poles (33.347, -635.7956) (33.5121, -635.804) (33.82, -635.8197) (34.0631, -636.0071) (34.1758, -636.094) knots 0 0 0 0 0.048244 0.08997 0.08997 0.08997 0.08997
  spline S881 degree 3 poles (34.1758, -636.094) (34.2601, -636.2163) (34.4495, -636.4912) (34.4599, -636.8269) (34.4657, -637.0132) knots 0 0 0 0 0.043695 0.098195 0.098195 0.098195 0.098195
  line L292 (34.4657, -637.0132) -> (34.4658, -639.4995)
  line L293 (34.4658, -639.4995) -> (33.8553, -639.4995)
  line L294 (33.8553, -639.4995) -> (33.8552, -637.2178)
  spline S882 degree 3 poles (33.8552, -637.2178) (33.8552, -637.1116) (33.8552, -636.9323) (33.8128, -636.7584) (33.7955, -636.6875) knots 0 0 0 0 0.031711 0.053535 0.053535 0.053535 0.053535
  spline S883 degree 3 poles (33.7955, -636.6875) (33.7711, -636.6358) (33.7212, -636.5304) (33.627, -636.4616) (33.5789, -636.4266) knots 0 0 0 0 0.016863 0.034394 0.034394 0.034394 0.034394
  spline S884 degree 3 poles (33.5789, -636.4266) (33.5232, -636.3977) (33.4078, -636.338) (33.2778, -636.3312) (33.2106, -636.3277) knots 0 0 0 0 0.018597 0.038532 0.038532 0.038532 0.038532
  spline S885 degree 3 poles (33.2106, -636.3277) (33.0895, -636.3375) (32.8515, -636.3567) (32.6669, -636.5077) (32.5762, -636.5818) knots 0 0 0 0 0.035532 0.069798 0.069798 0.069798 0.069798
  spline S886 degree 3 poles (32.5762, -636.5818) (32.5029, -636.6885) (32.3358, -636.9316) (32.3281, -637.2286) (32.3239, -637.3952) knots 0 0 0 0 0.038079 0.086792 0.086792 0.086792 0.086792
  line L295 (32.3239, -637.3952) -> (32.3239, -639.4996)
  line L296 (32.3239, -639.4996) -> (31.71, -639.4996)
  line L297 (31.71, -639.4996) -> (31.7099, -637.1462)
  spline S887 degree 3 poles (31.7099, -637.1462) (31.7075, -637.0242) (31.7032, -636.8074) (31.6034, -636.616) (31.5598, -636.5323) knots 0 0 0 0 0.036008 0.063954 0.063954 0.063954 0.063954
  spline S888 degree 3 poles (31.5598, -636.5323) (31.4976, -636.4728) (31.3614, -636.3424) (31.1717, -636.3329) (31.0687, -636.3277) knots 0 0 0 0 0.025037 0.054812 0.054812 0.054812 0.054812
  spline S889 degree 3 poles (31.0687, -636.3277) (30.984, -636.3334) (30.8145, -636.3447) (30.6645, -636.4244) (30.5895, -636.4642) knots 0 0 0 0 0.025172 0.050327 0.050327 0.050327 0.050327
  spline S890 degree 3 poles (30.5895, -636.4642) (30.5209, -636.5158) (30.3806, -636.6214) (30.3078, -636.7814) (30.2706, -636.8632) knots 0 0 0 0 0.025339 0.051812 0.051812 0.051812 0.051812
  spline S891 degree 3 poles (30.2706, -636.8632) (30.2419, -636.9695) (30.1751, -637.2171) (30.173, -637.4738) (30.1717, -637.6204) knots 0 0 0 0 0.032907 0.076633 0.076633 0.076633 0.076633
  line L298 (30.1717, -637.6204) -> (30.1718, -639.4996)
  line L299 (30.1718, -639.4996) -> (29.5579, -639.4997)
  line L300 (21.3519, -638.9098) -> (21.3519, -639.4999)
  line L301 (21.3519, -639.4999) -> (18.047, -639.5)
  spline S892 degree 3 poles (18.047, -639.5) (18.0482, -639.4269) (18.0507, -639.2812) (18.096, -639.1427) (18.1186, -639.0736) knots 0 0 0 0 0.021791 0.043448 0.043448 0.043448 0.043448
  spline S893 degree 3 poles (18.1186, -639.0736) (18.1689, -638.9593) (18.2742, -638.7199) (18.4374, -638.5154) (18.5227, -638.4086) knots 0 0 0 0 0.037314 0.078118 0.078118 0.078118 0.078118
  spline S894 degree 3 poles (18.5227, -638.4086) (18.6338, -638.2886) (18.8843, -638.0181) (19.168, -637.7825) (19.3259, -637.6514) knots 0 0 0 0 0.048996 0.110487 0.110487 0.110487 0.110487
  spline S895 degree 3 poles (19.3259, -637.6514) (19.5606, -637.4589) (19.9561, -637.1347) (20.2913, -636.7491) (20.4275, -636.5923) knots 0 0 0 0 0.090844 0.153043 0.153043 0.153043 0.153043
  spline S896 degree 3 poles (20.4275, -636.5923) (20.5109, -636.4701) (20.6641, -636.2454) (20.6984, -635.9765) (20.714, -635.8539) knots 0 0 0 0 0.043642 0.080205 0.080205 0.080205 0.080205
  spline S897 degree 3 poles (20.714, -635.8539) (20.7032, -635.7371) (20.6817, -635.5041) (20.5292, -635.3268) (20.4531, -635.2383) knots 0 0 0 0 0.034264 0.068363 0.068363 0.068363 0.068363
  spline S898 degree 3 poles (20.4531, -635.2383) (20.3568, -635.1652) (20.156, -635.0128) (19.9039, -634.9963) (19.7726, -634.9876) knots 0 0 0 0 0.035452 0.073952 0.073952 0.073952 0.073952
  spline S899 degree 3 poles (19.7726, -634.9876) (19.6345, -634.9965) (19.3704, -635.0136) (19.1624, -635.1761) (19.0632, -635.2537) knots 0 0 0 0 0.040455 0.077352 0.077352 0.077352 0.077352
  spline S900 degree 3 poles (19.0632, -635.2537) (18.9855, -635.3553) (18.8198, -635.572) (18.8028, -635.8452) (18.7938, -635.9904) knots 0 0 0 0 0.037518 0.080034 0.080034 0.080034 0.080034
  line L302 (18.7938, -635.9904) -> (18.1628, -635.9256)
  spline S901 degree 3 poles (18.1628, -635.9256) (18.1943, -635.7089) (18.2535, -635.3018) (18.524, -634.9937) (18.6505, -634.8495) knots 0 0 0 0 0.064088 0.120417 0.120417 0.120417 0.120417
  spline S902 degree 3 poles (18.6505, -634.8495) (18.8105, -634.7417) (19.1526, -634.5111) (19.5661, -634.4904) (19.7863, -634.4795) knots 0 0 0 0 0.056784 0.121484 0.121484 0.121484 0.121484
  spline S903 degree 3 poles (19.7863, -634.4795) (20.0088, -634.4917) (20.4285, -634.5147) (20.7666, -634.7622) (20.9254, -634.8785) knots 0 0 0 0 0.065229 0.123034 0.123034 0.123034 0.123034
  spline S904 degree 3 poles (20.9254, -634.8785) (21.0478, -635.02) (21.2938, -635.3045) (21.3278, -635.6792) (21.345, -635.8675) knots 0 0 0 0 0.054646 0.10988 0.10988 0.10988 0.10988
  spline S905 degree 3 poles (21.345, -635.8675) (21.3396, -635.9677) (21.3287, -636.1706) (21.258, -636.3612) (21.2222, -636.4576) knots 0 0 0 0 0.029916 0.060578 0.060578 0.060578 0.060578
  spline S906 degree 3 poles (21.2222, -636.4576) (21.1713, -636.5591) (21.0608, -636.7793) (20.9009, -636.9669) (20.8146, -637.0681) knots 0 0 0 0 0.033943 0.073642 0.073642 0.073642 0.073642
  spline S907 degree 3 poles (20.8146, -637.0681) (20.69, -637.1966) (20.3897, -637.5062) (20.0606, -637.785) (19.8682, -637.9481) knots 0 0 0 0 0.05369 0.129298 0.129298 0.129298 0.129298
  spline S908 degree 3 poles (19.8682, -637.9481) (19.7151, -638.0758) (19.4723, -638.2784) (19.2434, -638.4966) (19.1588, -638.5774) knots 0 0 0 0 0.059772 0.09485 0.09485 0.09485 0.09485
  spline S909 degree 3 poles (19.1588, -638.5774) (19.1095, -638.6314) (19.0145, -638.7356) (18.9369, -638.8533) (18.8996, -638.9099) knots 0 0 0 0 0.021914 0.042221 0.042221 0.042221 0.042221
  line L303 (18.8996, -638.9099) -> (21.3519, -638.9098)
  line L304 (29.2783, -689.4998) -> (29.2783, -685.8777)
  line L305 (29.2783, -685.8777) -> (29.8274, -685.8777)
  line L306 (29.8274, -685.8777) -> (29.8274, -686.3859)
  spline S910 degree 3 poles (29.8274, -686.3859) (29.8893, -686.3014) (30.0142, -686.1308) (30.1916, -686.0158) (30.281, -685.9579) knots 0 0 0 0 0.031158 0.062835 0.062835 0.062835 0.062835
  spline S911 degree 3 poles (30.281, -685.9579) (30.3802, -685.9106) (30.5841, -685.8135) (30.8097, -685.8019) (30.9256, -685.7959) knots 0 0 0 0 0.032617 0.067048 0.067048 0.067048 0.067048
  spline S912 degree 3 poles (30.9256, -685.7959) (31.0501, -685.8006) (31.2825, -685.8095) (31.4895, -685.9143) (31.5856, -685.963) knots 0 0 0 0 0.036859 0.068796 0.068796 0.068796 0.068796
  spline S913 degree 3 poles (31.5856, -685.963) (31.6652, -686.0247) (31.8262, -686.1494) (31.9077, -686.336) (31.9488, -686.4302) knots 0 0 0 0 0.029725 0.060035 0.060035 0.060035 0.060035
  spline S914 degree 3 poles (31.9488, -686.4302) (32.099, -686.2453) (32.3901, -685.8867) (32.8465, -685.8255) (33.0675, -685.7958) knots 0 0 0 0 0.068625 0.133023 0.133023 0.133023 0.133023
  spline S915 degree 3 poles (33.0675, -685.7958) (33.2326, -685.8042) (33.5405, -685.8199) (33.7835, -686.0073) (33.8963, -686.0943) knots 0 0 0 0 0.048244 0.08997 0.08997 0.08997 0.08997
  spline S916 degree 3 poles (33.8963, -686.0943) (33.9806, -686.2166) (34.17, -686.4915) (34.1804, -686.8271) (34.1862, -687.0134) knots 0 0 0 0 0.043695 0.098195 0.098195 0.098195 0.098195
  line L307 (34.1862, -687.0134) -> (34.1862, -689.4998)
  line L308 (34.1862, -689.4998) -> (33.5757, -689.4998)
  line L309 (33.5757, -689.4998) -> (33.5757, -687.2181)
  spline S917 degree 3 poles (33.5757, -687.2181) (33.5757, -687.1119) (33.5756, -686.9325) (33.5333, -686.7586) (33.516, -686.6877) knots 0 0 0 0 0.031711 0.053535 0.053535 0.053535 0.053535
  spline S918 degree 3 poles (33.516, -686.6877) (33.4916, -686.636) (33.4417, -686.5306) (33.3475, -686.4619) (33.2994, -686.4268) knots 0 0 0 0 0.016863 0.034394 0.034394 0.034394 0.034394
  spline S919 degree 3 poles (33.2994, -686.4268) (33.2437, -686.398) (33.1283, -686.3382) (32.9983, -686.3314) (32.9311, -686.3279) knots 0 0 0 0 0.018597 0.038532 0.038532 0.038532 0.038532
  spline S920 degree 3 poles (32.9311, -686.3279) (32.8099, -686.3377) (32.572, -686.357) (32.3873, -686.5079) (32.2967, -686.582) knots 0 0 0 0 0.035532 0.069798 0.069798 0.069798 0.069798
  spline S921 degree 3 poles (32.2967, -686.582) (32.2234, -686.6887) (32.0562, -686.9319) (32.0486, -687.2288) (32.0443, -687.3954) knots 0 0 0 0 0.038079 0.086792 0.086792 0.086792 0.086792
  line L310 (32.0443, -687.3954) -> (32.0443, -689.4998)
  line L311 (32.0443, -689.4998) -> (31.4304, -689.4998)
  line L312 (31.4304, -689.4998) -> (31.4304, -687.1465)
  spline S922 degree 3 poles (31.4304, -687.1465) (31.428, -687.0244) (31.4237, -686.8076) (31.3239, -686.6162) (31.2803, -686.5326) knots 0 0 0 0 0.036008 0.063954 0.063954 0.063954 0.063954
  spline S923 degree 3 poles (31.2803, -686.5326) (31.2181, -686.473) (31.0819, -686.3426) (30.8922, -686.3331) (30.7892, -686.3279) knots 0 0 0 0 0.025037 0.054812 0.054812 0.054812 0.054812
  spline S924 degree 3 poles (30.7892, -686.3279) (30.7044, -686.3336) (30.535, -686.345) (30.385, -686.4246) (30.31, -686.4644) knots 0 0 0 0 0.025173 0.050327 0.050327 0.050327 0.050327
  spline S925 degree 3 poles (30.31, -686.4644) (30.2414, -686.516) (30.1011, -686.6216) (30.0283, -686.7817) (29.9911, -686.8634) knots 0 0 0 0 0.025339 0.051812 0.051812 0.051812 0.051812
  spline S926 degree 3 poles (29.9911, -686.8634) (29.9624, -686.9697) (29.8956, -687.2173) (29.8934, -687.474) (29.8922, -687.6206) knots 0 0 0 0 0.032907 0.076633 0.076633 0.076633 0.076633
  line L313 (29.8922, -687.6206) -> (29.8922, -689.4998)
  line L314 (29.8922, -689.4998) -> (29.2783, -689.4998)
  line L315 (20.1583, -689.5) -> (19.5443, -689.5)
  line L316 (19.5443, -689.5) -> (19.5443, -685.588)
  spline S927 degree 3 poles (19.5443, -685.588) (19.4606, -685.6608) (19.2792, -685.8187) (19.0736, -685.9436) (18.9628, -686.0109) knots 0 0 0 0 0.033221 0.072019 0.072019 0.072019 0.072019